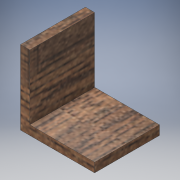
# Autodesk Inventor part: Post Bracket
Saved by Autodesk Inventor 2017 (Build 210142000, 142)
## iProperties
Created: 2016-09-08
Part Number: Post Bracket
Material: Generic
Document SubType Name: Modeling
Designer: s.ethan.wierenga
Density: 1 g/cm^3
Appearance: White Ash - Java
Author: s.ethan.wierenga
Autodesk Inventor part; units mm, degrees
ref_plane "YZ Plane" through (0, 0, 0) normal (1, 0, 0) x (0, 1, 0)
ref_plane "XZ Plane" through (0, 0, 0) normal (0, 1, 0) x (-1, 0, 0)
ref_plane "XY Plane" through (0, 0, 0) normal (0, 0, 1) x (1, 0, 0)
sketch "Sketch1" plane through (0, 0, 0) normal (0, 1, 0) x (-1, 0, 0)
  line L0 (0, 0) -> (0, -88.9)
  line L1 (0, -88.9) -> (-101.6, -88.9)
  line L2 (-101.6, -88.9) -> (-101.6, 0)
  line L3 (-101.6, 0) -> (0, 0)
  dimension "d0" = 88.9
  dimension "d1" = 101.6
  constraints: 8 end point, 3 perpendicular, 1 vertical
  measures "d0" distance of L0.start L0.end
  measures "d1" distance of L0.end L1.end
extrude "Extrusion1" add sketch "Sketch1" along normal blind 12.7
sketch "Sketch2" plane through (0, 12.7, 0) normal (0, 1, 0) x (1, 0, 0)
  line L0 (101.6, 88.9) -> (0, 88.9) projected
  line L1 (0, 0) -> (12.7, 0)
  line L2 (12.7, 0) -> (12.7, 88.9)
  line L3 (12.7, 88.9) -> (0, 88.9)
  line L4 (0, 88.9) -> (0, 0)
  dimension "d4" = 12.7
  constraints: 8 end point, 2 parallel, 1 horizontal, 1 perpendicular, 1 point on line
  measures "d4" distance of L3.end L2.end
extrude "Extrusion2" add sketch "Sketch2" along normal blind 88.9
body "Solid1"
